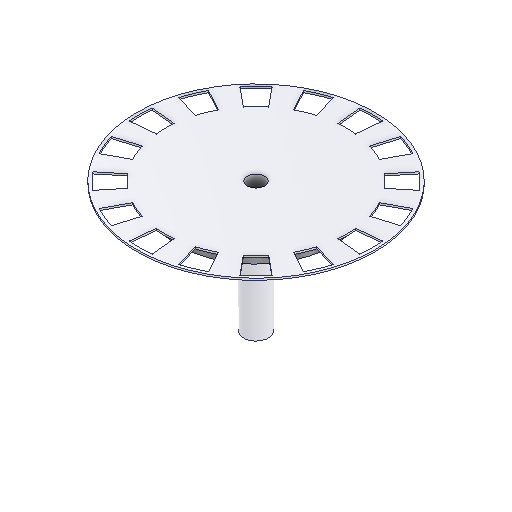
# Autodesk Inventor part: Eje_econder
Saved by Autodesk Inventor 2025.2 (Build 292293000, 293)
## iProperties
Created: 2025-05-05
Part Number: Eje_econder
Material: PET Plastic
Document SubType Name: Modeling
Designer: nicoa
Density: 1.541 g/cm^3
Appearance: PTFE
Mass: 10.298 g
Surface Area: 109.925 cm^2
Volume: 6.6827 cm^3
Author: nicoa
Autodesk Inventor part; units mm, degrees
ref_plane "YZ Plane" through (0, 0, 0) normal (1, 0, 0) x (0, 1, 0)
ref_plane "XZ Plane" through (0, 0, 0) normal (0, 1, 0) x (-1, 0, 0)
ref_plane "XY Plane" through (0, 0, 0) normal (0, 0, 1) x (1, 0, 0)
sketch "Sketch1" plane through (0, 0, 0) normal (0, 1, 0) x (-1, 0, 0)
  circle A0 centre (0, 0) radius 4.0309
  circle A1 centre (0, 0) radius 3.3
  dimension "d0" = 6.6
  constraints: 2 centre point, 2 coincident
  measures "d0" diameter of A1
extrude "Extrusion1" add sketch "Sketch1" along normal blind 42
sketch "Sketch2" plane through (0, 42, 0) normal (0, 1, 0) x (1, 0, 0)
  circle A0 centre (0, 0) radius 4.0309 projected
  circle A1 centre (0, 0) radius 3.3 projected
  circle A2 centre (0, 0) radius 2.8
  dimension "d3" = 5.6
  constraints: 1 centre point, 1 coincident
  measures "d3" diameter of A2
extrude "Extrusion2" add sketch "Sketch2" against normal blind 5 contours A1
sketch "Sketch3" plane through (0, 42, 0) normal (0, 1, 0) x (1, 0, 0)
  circle A0 centre (0, 0) radius 38.5
  circle A1 centre (0, 0) radius 25
  circle A2 centre (0, 0) radius 4.0309 projected
  circle A3 centre (0, 0) radius 2.8 projected
  line L0 (0, 4.0309) -> (38.2884, 4.0309)
  line L1 (0, -4.0309) -> (38.2884, -4.0309)
  line L2 (-3.4908, -2.0154) -> (-22.635, 31.1433)
  line L3 (3.4908, 2.0154) -> (-15.6534, 35.1742)
  line L4 (3.4908, -2.0154) -> (-15.6534, -35.1742)
  line L5 (-3.4908, 2.0154) -> (-22.635, -31.1433)
  point P0 (24.6729, 4.0309)
  point P1 (24.6729, -4.0309)
  point P2 (-4.6544, 0)
  point P3 (-3.4908, 2.0154)
  point P4 (2.3272, 4.0309)
  point P5 (-8.8456, 23.3828)
  point P6 (-15.8273, 19.3519)
  point P7 (-15.8273, -19.3519)
  point P8 (-8.8456, -23.3828)
  point P9 (2.3272, -4.0309)
  point P10 (-3.4908, -2.0154)
  point P11 (-22.635, -31.1433)
  point P12 (-22.635, 31.1433)
  point P13 (3.4908, -2.0154)
  point P14 (-15.6534, -35.1742)
  point P15 (-15.6534, 35.1742)
  dimension "d10" = 77
  dimension "d11" = 50
  dimension "d28" = 360
  constraints: 12 end point, 4 point on circle, 2 centre point, 2 coincident, 1 horizontal, 1 parallel, 1 tangent, 19 other
  measures "d10" diameter of A0
  measures "d11" diameter of A1
extrude "Extrusion3" add sketch "Sketch3" against normal blind 0.6 contours A0 L1 A1 L0 | L0 A1 L3 A0 | A0 L4 A1 L1 | L3 A1 L2 A0 | L0 L3 A1 | A1 L1 L4 A2 L3 L0 | A0 L5 A1 L4 | A1 L4 L1 | L2 A1 L5 A0 | L3 L0 A2 L5 L2 A1 | L3 A2 L0 | A1 L5 L2 A2 L1 L4 | L1 A2 L4 | L2 L5 A1 | A2 | L5 A2 L2 | A3
fillet "Fillet1" [suppressed]
sketch "Sketch4" plane through (0, 42, 0) normal (0, 1, 0) x (1, 0, 0)
  circle A0 centre (0, 0) radius 39.5 projected
  circle A1 centre (0, 0) radius 37.5
  circle A2 centre (0, 0) radius 29.5
  line L0 (-39.5, 0) -> (0, 0)
  line L1 (0, 0) -> (-37.3194, 3.6756)
  line L2 (0, 0) -> (-37.3194, -3.6756)
  line L3 (0, 0) -> (-35.8853, -10.8857)
  line L4 (0, 0) -> (-33.072, -17.6774)
  line L5 (0, 0) -> (-28.9879, -23.7897)
  line L6 (0, 0) -> (-23.7897, -28.9879)
  line L7 (0, 0) -> (-17.6774, -33.072)
  line L8 (0, 0) -> (-10.8857, -35.8853)
  line L9 (0, 0) -> (-3.6756, -37.3194)
  line L10 (0, 0) -> (3.6756, -37.3194)
  line L11 (0, 0) -> (10.8857, -35.8853)
  line L12 (0, 0) -> (17.6774, -33.072)
  line L13 (0, 0) -> (23.7897, -28.9879)
  line L14 (0, 0) -> (28.9879, -23.7897)
  line L15 (0, 0) -> (33.072, -17.6774)
  line L16 (0, 0) -> (35.8853, -10.8857)
  line L17 (0, 0) -> (37.3194, -3.6756)
  line L18 (0, 0) -> (37.3194, 3.6756)
  line L19 (0, 0) -> (35.8853, 10.8857)
  line L20 (0, 0) -> (33.072, 17.6774)
  line L21 (0, 0) -> (28.9879, 23.7897)
  line L22 (0, 0) -> (23.7897, 28.9879)
  line L23 (0, 0) -> (17.6774, 33.072)
  line L24 (0, 0) -> (10.8857, 35.8853)
  line L25 (0, 0) -> (3.6756, 37.3194)
  line L26 (0, 0) -> (-3.6756, 37.3194)
  line L27 (0, 0) -> (-10.8857, 35.8853)
  line L28 (0, 0) -> (-17.6774, 33.072)
  line L29 (0, 0) -> (-23.7897, 28.9879)
  line L30 (0, 0) -> (-28.9879, 23.7897)
  line L31 (0, 0) -> (-33.072, 17.6774)
  line L32 (0, 0) -> (-35.8853, 10.8857)
  point P0 (-23.7897, -28.9879)
  point P1 (-18.7146, -22.8038)
  point P2 (-22.8038, -18.7146)
  point P3 (-28.9879, -23.7897)
  point P4 (-10.8857, -35.8853)
  point P5 (-8.5634, -28.2297)
  point P6 (-13.9062, -26.0167)
  point P7 (-17.6774, -33.072)
  point P8 (3.6756, -37.3194)
  point P9 (2.8915, -29.3579)
  point P10 (-2.8915, -29.3579)
  point P11 (17.6774, -33.072)
  point P12 (13.9062, -26.0167)
  point P13 (8.5634, -28.2297)
  point P14 (10.8857, -35.8853)
  point P15 (28.9879, -23.7897)
  point P16 (22.8038, -18.7146)
  point P17 (18.7146, -22.8038)
  point P18 (23.7897, -28.9879)
  point P19 (35.8853, -10.8857)
  point P20 (28.2297, -8.5634)
  point P21 (26.0167, -13.9062)
  point P22 (33.072, -17.6774)
  point P23 (-33.072, -17.6774)
  point P24 (-26.0167, -13.9062)
  point P25 (-28.2297, -8.5634)
  point P26 (-35.8853, -10.8857)
  point P27 (-29.3579, -2.8915)
  point P28 (-29.3579, 2.8915)
  point P29 (37.3194, 3.6756)
  point P30 (29.3579, 2.8915)
  point P31 (29.3579, -2.8915)
  point P32 (37.3194, -3.6756)
  point P33 (33.072, 17.6774)
  point P34 (26.0167, 13.9062)
  point P35 (28.2297, 8.5634)
  point P36 (35.8853, 10.8857)
  point P37 (23.7897, 28.9879)
  point P38 (18.7146, 22.8038)
  point P39 (22.8038, 18.7146)
  point P40 (28.9879, 23.7897)
  point P41 (10.8857, 35.8853)
  point P42 (8.5634, 28.2297)
  point P43 (13.9062, 26.0167)
  point P44 (17.6774, 33.072)
  point P45 (-3.6756, 37.3194)
  point P46 (-2.8915, 29.3579)
  point P47 (2.8915, 29.3579)
  point P48 (3.6756, 37.3194)
  point P49 (-17.6774, 33.072)
  point P50 (-13.9062, 26.0167)
  point P51 (-8.5634, 28.2297)
  point P52 (-10.8857, 35.8853)
  point P53 (-35.8853, 10.8857)
  point P54 (-28.2297, 8.5634)
  point P55 (-26.0167, 13.9062)
  point P56 (-33.072, 17.6774)
  point P57 (-28.9879, 23.7897)
  point P58 (-22.8038, 18.7146)
  point P59 (-18.7146, 22.8038)
  point P60 (-23.7897, 28.9879)
  dimension "d15" = 2
  dimension "d16" = 8
  dimension "d17" = 5.625
  dimension "d19" = 5.625
  dimension "d22" = 360
  constraints: 66 end point, 1 horizontal, 1 horizontal alignment, 88 other
  measures "d17" angle of L0 L1
  measures "d19" angle of L0 L2
extrude "Extrusion4" cut sketch "Sketch4" against normal through all contours A1 L1 A2 L0 | L0 A2 L2 A1 | A1 L31 A2 L32 | L3 A2 L4 A1 | A2 L6 A1 L5 | A2 L8 A1 L7 | A2 L10 A1 L9 | A2 L12 A1 L11 | A2 L14 A1 L13 | A2 L16 A1 L15 | A2 L18 A1 L17 | A2 L20 A1 L19 | A2 L22 A1 L21 | A2 L24 A1 L23 | A2 L26 A1 L25 | A2 L28 A1 L27 | A2 L30 A1 L29
fillet "Fillet2" [suppressed]
sketch "Sketch5" plane through (0, 41.4, 0) normal (0, -1, 0) x (1, 0, 0)
  circle A0 centre (0, 0) radius 2.8 projected
extrude "Extrusion5" cut sketch "Sketch5" against normal blind 0.6
fillet "Fillet3" radius 2 1 edges at (4.0309, 41.4, 0)
sketch "Sketch6" plane through (0, 41.4, 0) normal (0, -1, 0) x (1, 0, 0)
  circle A0 centre (0, 0) radius 25
  circle A1 centre (0, 0) radius 4.0309 projected
  circle A2 centre (0, 0) radius 22.5
  dimension "d34" = 50
  dimension "d35" = 45
  constraints: 2 centre point, 2 coincident
  measures "d34" diameter of A0
  measures "d35" diameter of A2
extrude "Extrusion6" add sketch "Sketch6" along normal blind 5 contours A0
fillet "Fillet4" radius 1 2 edges at (-22.5, 41.4, 0) (-25, 41.4, 0)
body "Solid1"
